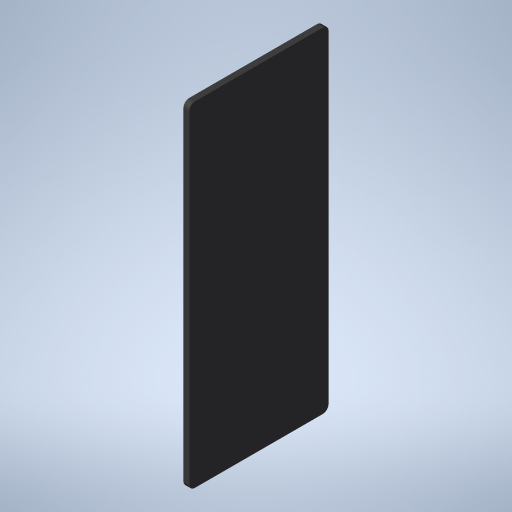
# Autodesk Inventor part: ChamberSides
Saved by Autodesk Inventor 2023 (Build 270158000, 158)
## iProperties
Created: 2025-11-21
Part Number: ChamberSides
Material: Generic
Document SubType Name: Modeling
Designer: DanAr
Density: 1 g/cm^3
Appearance: Default
Author: DanAr
Autodesk Inventor part; units mm, degrees
ref_plane "YZ Plane" through (0, 0, 0) normal (1, 0, 0) x (0, 1, 0)
ref_plane "XZ Plane" through (0, 0, 0) normal (0, 1, 0) x (-1, 0, 0)
ref_plane "XY Plane" through (0, 0, 0) normal (0, 0, 1) x (1, 0, 0)
sketch "Sketch1" plane through (0, 0, 0) normal (1, 0, 0) x (0, 1, 0)
  line L0 (0, 0) -> (179.8, 0)
  line L1 (179.8, 0) -> (179.8, -74.8)
  line L2 (179.8, -74.8) -> (0, -74.8)
  line L3 (0, -74.8) -> (0, 0)
  dimension "d0" = 179.8
  dimension "d1" = 74.8
  constraints: 8 end point, 2 parallel, 1 horizontal, 1 perpendicular
  measures "d0" distance of L1.end L2.end
  measures "d1" distance of L0.end L1.end
extrude "Extrusion1" add sketch "Sketch1" along normal blind 3
fillet "Fillet1" radius 3 4 edges at (1.5, 179.8, 0) (1.5, 179.8, -74.8) (1.5, 0, 0) (1.5, 0, -74.8)
body "Solid1"
